Autodesk Fusion 360 part; units mm, degrees
(part 2 of 2)
equation "d393_1 = 1.6 mm + 0.2 mm"
equation "d394_1 = d393_1 / 2"
named bodies: "Board", "Right", "Left", "Bottom", "Knob", "Top", "Right With Hole"
